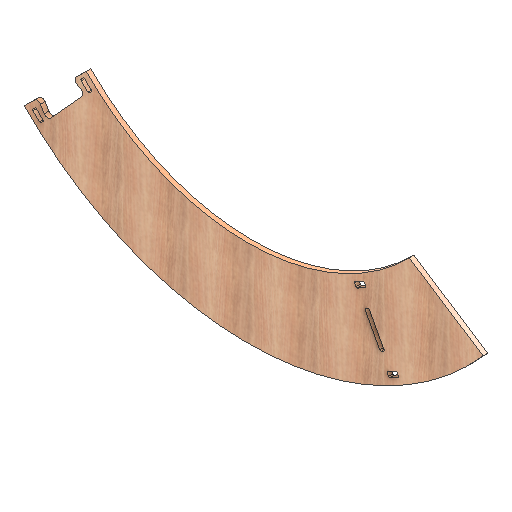
# Autodesk Inventor part: Platform E4
Saved by Autodesk Inventor 2021 (Build 250183000, 183)
## iProperties
Created: 2020-05-09
Part Number: Platform E4
Material: Wood (Birch)
Document SubType Name: Modeling
Designer: Dan Wikman
Density: 0.55 g/cm^3
Appearance: Birch - Natural Polished
Mass: 5520.25 g
Surface Area: 12045.4 cm^2
Volume: 10036.8 cm^3
Autodesk Inventor part; units mm, degrees
ref_plane "YZ Plane" through (0, 0, 0) normal (1, 0, 0) x (0, 1, 0)
ref_plane "XZ Plane" through (0, 0, 0) normal (0, 1, 0) x (-1, 0, 0)
ref_plane "XY Plane" through (0, 0, 0) normal (0, 0, 1) x (1, 0, 0)
sketch "CONTOURS" plane through (0, 0, 0) normal (0, 0, 1) x (1, 0, 0)
  arc A0 (28.0046, 396.7552) -> (1814.0653, 446.8716) centre (897.7889, 1250.2638) ccw
  line L0 (28.0046, 396.7552) -> (68.5769, 436.5356)
  arc A1 (91.1499, 433.6624) -> (68.5769, 436.5356) centre (78.7284, 426.182) ccw
  line L1 (91.1499, 433.6624) -> (106.0415, 408.9341)
  arc A2 (106.0415, 408.9341) -> (130.7846, 406.4993) centre (119.3197, 416.9304) ccw
  line L2 (130.7846, 406.4993) -> (251.8873, 539.6044)
  arc A3 (251.8873, 539.6044) -> (247.9235, 563.5995) centre (240.4224, 550.0355) ccw
  line L3 (247.9235, 563.5995) -> (233.1425, 571.7736)
  arc A4 (230.0082, 594.8161) -> (233.1425, 571.7736) centre (240.1597, 584.4626) ccw
  line L4 (230.0082, 594.8161) -> (269.3503, 633.3904)
  arc A5 (269.3503, 633.3904) -> (1526.2271, 633.3904) centre (897.7887, 1250.4881) ccw
  line L5 (1526.2271, 633.3904) -> (1814.0653, 446.8716)
  constraints: 12 end point, 12 point on circle, 6 centre point
sketch "HOLES" plane through (0, 0, 0) normal (0, 0, 1) x (1, 0, 0)
  arc A0 (288.9886, 574.6199) -> (288.8907, 580.2759) centre (286.1117, 577.3989) ccw
  line L0 (288.9886, 574.6199) -> (281.3462, 566.7082)
  arc A1 (275.6902, 566.6103) -> (281.3462, 566.7082) centre (278.4693, 569.4873) ccw
  line L1 (275.6902, 566.6103) -> (249.7976, 591.6217)
  arc A2 (249.6997, 597.2778) -> (249.7976, 591.6217) centre (252.5767, 594.4987) ccw
  line L2 (1440.2918, 203.0579) -> (1445.4546, 193.3448)
  arc A3 (1445.4546, 193.3448) -> (1450.864, 191.6901) centre (1448.9867, 195.2221) ccw
  line L3 (1450.864, 191.6901) -> (1482.6526, 208.5865)
  arc A4 (1482.6526, 208.5865) -> (1484.3073, 213.9959) centre (1480.7752, 212.1185) ccw
  line L4 (1484.3073, 213.9959) -> (1479.1445, 223.7091)
  arc A5 (1479.1445, 223.7091) -> (1473.735, 225.3638) centre (1475.6124, 221.8317) ccw
  line L5 (1473.735, 225.3638) -> (1441.9465, 208.4674)
  arc A6 (1441.9465, 208.4674) -> (1440.2918, 203.0579) centre (1443.8239, 204.9353) ccw
  line L6 (101.125, 380.1374) -> (93.4826, 372.2258)
  arc A7 (87.8266, 372.1279) -> (93.4826, 372.2258) centre (90.6056, 375.0048) ccw
  line L7 (87.8266, 372.1279) -> (61.9339, 397.1393)
  arc A8 (61.836, 402.7953) -> (61.9339, 397.1393) centre (64.713, 400.0162) ccw
  line L8 (61.836, 402.7953) -> (69.4784, 410.7069)
  arc A9 (75.1344, 410.8048) -> (69.4784, 410.7069) centre (72.3554, 407.9279) ccw
  line L9 (75.1344, 410.8048) -> (101.027, 385.7934)
  arc A10 (101.125, 380.1374) -> (101.027, 385.7934) centre (98.248, 382.9165) ccw
  line L10 (1362.2188, 382.0722) -> (1356.0415, 378.7797)
  arc A11 (1356.0415, 378.7797) -> (1354.3929, 373.3684) centre (1357.9229, 375.2498) ccw
  line L11 (1354.3929, 373.3684) -> (1411.7752, 265.7057)
  arc A12 (1411.7752, 265.7057) -> (1417.1866, 264.0571) centre (1415.3052, 267.587) ccw
  line L12 (1417.1866, 264.0571) -> (1426.8939, 269.2309)
  arc A13 (1426.8939, 269.2309) -> (1428.5424, 274.6423) centre (1425.0125, 272.7609) ccw
  line L13 (1428.5424, 274.6423) -> (1371.1601, 382.305)
  arc A14 (1371.1601, 382.305) -> (1365.7488, 383.9536) centre (1367.6302, 380.4236) ccw
  line L14 (1365.7488, 383.9536) -> (1362.2188, 382.0722)
  line L15 (249.6997, 597.2778) -> (257.3421, 605.1894)
  arc A15 (262.9981, 605.2873) -> (257.3421, 605.1894) centre (260.219, 602.4103) ccw
  line L16 (262.9981, 605.2873) -> (288.8907, 580.2759)
  line L17 (1318.5439, 432.1121) -> (1313.3811, 441.8253)
  arc A16 (1315.0357, 447.2347) -> (1313.3811, 441.8253) centre (1316.9131, 443.7027) ccw
  line L18 (1315.0357, 447.2347) -> (1346.8243, 464.1311)
  arc A17 (1352.2337, 462.4764) -> (1346.8243, 464.1311) centre (1348.7017, 460.5991) ccw
  line L19 (1352.2337, 462.4764) -> (1357.3965, 452.7633)
  arc A18 (1355.7418, 447.3538) -> (1357.3965, 452.7633) centre (1353.8645, 450.8859) ccw
  line L20 (1355.7418, 447.3538) -> (1323.9533, 430.4574)
  arc A19 (1318.5439, 432.1121) -> (1323.9533, 430.4574) centre (1322.0759, 433.9895) ccw
  constraints: 42 end point, 40 point on circle, 20 centre point
sketch "LETTERS" plane through (0, 0, 0) normal (0, 0, 1) x (1, 0, 0)
  line L0 (243.6817, 427.6795) -> (251.9783, 420.9747)
  line L1 (249.8017, 435.2055) -> (237.3515, 419.7995)
  line L2 (237.3515, 419.7995) -> (248.775, 410.5677)
  line L3 (261.2252, 425.9736) -> (249.8017, 435.2055)
  constraints: 8 end point, 2 parallel, 1 perpendicular
extrude "Extrusion1" add sketch "CONTOURS" along normal blind 18
extrude "Extrusion2" cut sketch "HOLES" along normal blind 18
body "Solid1"
